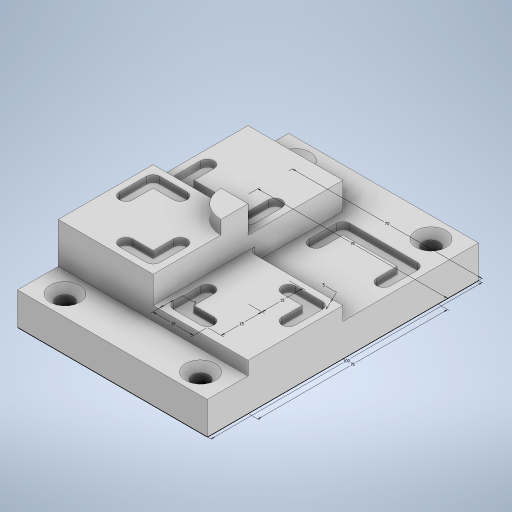
# Autodesk Inventor part: SmallTool20mm
Saved by Autodesk Inventor 2024 (Build 280153000, 153)
## iProperties
Created: 2026-02-22
Part Number: SmallTool20mm
Material: Generic
Document SubType Name: Modeling
Designer: Nathan
Density: 1 g/cm^3
Appearance: Default
Author: Nathan
Autodesk Inventor part; units mm, degrees
ref_plane "YZ Plane" through (0, 0, 0) normal (1, 0, 0) x (0, 1, 0)
ref_plane "XZ Plane" through (0, 0, 0) normal (0, 1, 0) x (-1, 0, 0)
ref_plane "XY Plane" through (0, 0, 0) normal (0, 0, 1) x (1, 0, 0)
sketch "Sketch1" plane through (0, 0, 0) normal (0, 1, 0) x (-1, 0, 0)
  line L0 (35, 50) -> (-35, 50)
  line L1 (-35, 50) -> (-35, -50)
  line L2 (-35, -50) -> (35, -50)
  line L3 (35, -50) -> (35, 50)
  line L4 (35, 50) -> (-35, -50) construction
  line L5 (-35, 50) -> (35, -50) construction
  line L6 (35, 35) -> (-35, 35)
  line L7 (-35, 35) -> (-35, -35)
  line L8 (-35, -35) -> (35, -35)
  line L9 (35, -35) -> (35, 35)
  line L10 (35, 35) -> (-35, -35) construction
  line L11 (-35, 35) -> (35, -35) construction
  line L12 (0, 35) -> (0, -35)
  line L13 (35, 0) -> (-35, 0)
  line L14 (0, 0) -> (0, 15) construction
  line L15 (0, 15) -> (15, 15) construction
  line L16 (0, 0) -> (0, -15) construction
  line L17 (0, -15) -> (-15, -15) construction
  circle A0 centre (15, 15) radius 2.5
  circle A1 centre (-15, -15) radius 2.5
  dimension "d0" = 70
  dimension "d1" = 100
  dimension "d2" = 70
  dimension "d3" = 70
  dimension "d46" = 15
  dimension "d47" = 15
  dimension "d48" = 15
  dimension "d49" = 5
  dimension "d50" = 5
  constraints: 36 end point, 8 midpoint, 4 parallel, 4 point on line, 3 perpendicular, 2 centre point, 2 coincident, 2 horizontal
  measures "d0" distance of L2.end L1.end
  measures "d1" distance of L1.end L0.end
  measures "d2" distance of L8.end L7.end
  measures "d3" distance of L7.end L6.end
  measures "d46" distance of L14.start L14.end
  measures "d47" distance of L14.end L15.end
  measures "d48" distance of L14.start L16.end
  measures "d49" diameter of A0
  measures "d50" diameter of A1
extrude "Extrusion1" add sketch "Sketch1" along normal blind 12 contours L3 L6 L1 L0 | L13 L12 L8 L1 | L3 L2 L1 L8 | A1
extrude "Extrusion2" add sketch "Sketch1" along normal blind 17 contours L6 L12 L13 L1
extrude "Extrusion3" add sketch "Sketch1" along normal blind 22 contours L3 L8 L12 L13
extrude "Extrusion4" add sketch "Sketch1" along normal blind 27 contours L3 L13 L12 L6 | A0
sketch "Sketch2" plane through (0, 27, 0) normal (0, 1, 0) x (1, 0, 0)
  line L0 (35, -35) -> (-35, -35) construction
  line L1 (35, 0) -> (0, 0) construction
  line L2 (-35, -35) -> (0, -35) construction
  line L3 (0, -35) -> (0, 0) construction
  line L4 (0, 0) -> (-35, 0) construction
  line L5 (-35, 0) -> (-35, -35) construction
  line L6 (0, -35) -> (-35, 0) construction
  line L7 (0, 0) -> (-35, -35) construction
  line L8 (-5, -32.5) -> (-15, -32.5)
  line L9 (-32.5, -15) -> (-32.5, -5)
  line L10 (-30, -2.5) -> (-20, -2.5)
  line L11 (-2.5, -20) -> (-2.5, -30)
  line L12 (-2.5, -32.5) -> (-32.5, -2.5) construction
  line L13 (-32.5, -32.5) -> (-2.5, -2.5) construction
  line L14 (-15, -27.5) -> (-10, -27.5)
  line L15 (-7.5, -25) -> (-7.5, -20)
  line L16 (-20, -7.5) -> (-25, -7.5)
  line L17 (-27.5, -10) -> (-27.5, -15)
  line L18 (-27.5, -27.5) -> (-7.5, -7.5) construction
  line L19 (-7.5, -27.5) -> (-27.5, -7.5) construction
  line L20 (-5, -17.5) -> (-5, -17.5)
  line L21 (-17.5, -30) -> (-17.5, -30)
  line L22 (-30, -17.5) -> (-30, -17.5)
  line L23 (-17.5, -5) -> (-17.5, -5)
  arc A0 (-17.5, -30) -> (-15, -32.5) centre (-15, -30) ccw
  arc A1 (-15, -27.5) -> (-17.5, -30) centre (-15, -30) ccw
  arc A2 (-5, -17.5) -> (-7.5, -20) centre (-5, -20) ccw
  arc A3 (-2.5, -20) -> (-5, -17.5) centre (-5, -20) ccw
  arc A4 (-5, -32.5) -> (-2.5, -30) centre (-5, -30) ccw
  arc A5 (-32.5, -15) -> (-30, -17.5) centre (-30, -15) ccw
  arc A6 (-30, -17.5) -> (-27.5, -15) centre (-30, -15) ccw
  arc A7 (-20, -7.5) -> (-17.5, -5) centre (-20, -5) ccw
  arc A8 (-17.5, -5) -> (-20, -2.5) centre (-20, -5) ccw
  arc A9 (-30, -2.5) -> (-32.5, -5) centre (-30, -5) ccw
  line L24 (5, -32.5) -> (15, -32.5)
  line L25 (32.5, -15) -> (32.5, -5)
  line L26 (30, -2.5) -> (20, -2.5)
  line L27 (2.5, -20) -> (2.5, -30)
  line L28 (15, -27.5) -> (10, -27.5)
  line L29 (7.5, -25) -> (7.5, -20)
  line L30 (20, -7.5) -> (25, -7.5)
  line L31 (27.5, -10) -> (27.5, -15)
  arc A10 (15, -32.5) -> (17.5, -30) centre (15, -30) ccw
  arc A11 (17.5, -30) -> (15, -27.5) centre (15, -30) ccw
  arc A12 (7.5, -20) -> (5, -17.5) centre (5, -20) ccw
  arc A13 (5, -17.5) -> (2.5, -20) centre (5, -20) ccw
  arc A14 (2.5, -30) -> (5, -32.5) centre (5, -30) ccw
  arc A15 (30, -17.5) -> (32.5, -15) centre (30, -15) ccw
  arc A16 (27.5, -15) -> (30, -17.5) centre (30, -15) ccw
  arc A17 (17.5, -5) -> (20, -7.5) centre (20, -5) ccw
  arc A18 (20, -2.5) -> (17.5, -5) centre (20, -5) ccw
  arc A19 (32.5, -5) -> (30, -2.5) centre (30, -5) ccw
  line L32 (7.5, 25) -> (7.5, 20)
  arc A20 (10, 27.5) -> (7.5, 25) centre (10, 25) ccw
  line L33 (15, 27.5) -> (10, 27.5)
  arc A21 (15, 27.5) -> (17.5, 30) centre (15, 30) ccw
  arc A22 (17.5, 30) -> (15, 32.5) centre (15, 30) ccw
  line L34 (5, 32.5) -> (15, 32.5)
  arc A23 (5, 32.5) -> (2.5, 30) centre (5, 30) ccw
  line L35 (2.5, 20) -> (2.5, 30)
  arc A24 (2.5, 20) -> (5, 17.5) centre (5, 20) ccw
  arc A25 (5, 17.5) -> (7.5, 20) centre (5, 20) ccw
  line L36 (-32.5, 15) -> (-32.5, 5)
  line L37 (-30, 2.5) -> (-20, 2.5)
  line L38 (-20, 7.5) -> (-25, 7.5)
  line L39 (-27.5, 10) -> (-27.5, 15)
  arc A26 (-30, 17.5) -> (-32.5, 15) centre (-30, 15) ccw
  arc A27 (-27.5, 15) -> (-30, 17.5) centre (-30, 15) ccw
  arc A28 (-27.5, 10) -> (-25, 7.5) centre (-25, 10) ccw
  arc A29 (-17.5, 5) -> (-20, 7.5) centre (-20, 5) ccw
  arc A30 (-20, 2.5) -> (-17.5, 5) centre (-20, 5) ccw
  arc A31 (-32.5, 5) -> (-30, 2.5) centre (-30, 5) ccw
  line L40 (-35, 50) -> (-35, 35) construction
  line L41 (35, -35) -> (35, 0) construction
  line L42 (-35, 35) -> (35, -35) construction
  line L43 (-10, -27.5) -> (-7.5, -27.5)
  line L44 (-7.5, -25) -> (-7.5, -27.5)
  line L45 (-27.5, -10) -> (-27.5, -7.5)
  line L46 (-27.5, -7.5) -> (-25, -7.5)
  line L47 (10, -27.5) -> (7.5, -27.5)
  line L48 (7.5, -27.5) -> (7.5, -25)
  line L49 (25, -7.5) -> (27.5, -7.5)
  line L50 (27.5, -7.5) -> (27.5, -10)
  point P0 (-17.5, -17.5)
  point P1 (-17.5, -17.5)
  point P2 (-7.5, -17.5)
  point P3 (-17.5, -27.5)
  point P4 (-17.5, -32.5)
  dimension "d12" = 30
  dimension "d13" = 30
  dimension "d16" = 15
  dimension "d17" = 5
  dimension "d18" = 10
  dimension "d19" = 10
  dimension "d20" = 2.5
  constraints: 94 end point, 68 symmetric about line, 64 point on circle, 32 centre point, 20 tangent, 14 point on line, 9 equal radius, 7 horizontal, 7 parallel, 7 perpendicular, 6 midpoint, 20 other
  measures "d12" distance of L12.end L13.end
  measures "d13" distance of L13.start L12.end
  measures "d16" distance of point (-17.5, -32.5) L12.start
  measures "d17" distance of point (-17.5, -27.5) point (-17.5, -32.5)
  measures "d18" distance of point (-17.5, -27.5) L19.start
  measures "d19" distance of point (-7.5, -17.5) L19.start
  measures "d20" radius of A0
fillet "Fillet1" radius 2.5 1 edges at (0, 14.5, 0)
extrude "Extrusion5" cut sketch "Sketch2" against normal blind 2.5 contours L8 A0 A1 L14 L43 L44 L15 A2 A3 L11 A4 | L9 A9 L10 A8 A7 L16 L46 L45 L17 A6 A5
extrude "Extrusion6" cut sketch "Sketch2" against normal blind 12.5 contours A14 L27 A13 A12 L29 L48 L47 L28 A11 A10 L24 | A15 A16 L31 L50 L49 L30 A17 A18 L26 A19 L25
sketch "Sketch3" plane through (0, 22, 0) normal (0, 1, 0) x (1, 0, 0)
  line L0 (0, 0) -> (0, 35) construction
  line L1 (-35, 50) -> (-35, -50) construction
  line L2 (0, 35) -> (-35, 35) construction
  line L3 (-35, 35) -> (-35, 0) construction
  line L4 (-35, 0) -> (0, 0) construction
  line L5 (0, 0) -> (0, 35) construction
  line L6 (-35, 35) -> (0, 0) construction
  line L7 (0, 35) -> (-35, 0) construction
  line L8 (-32.5, 15) -> (-32.5, 5)
  line L9 (-30, 2.5) -> (-5, 2.5)
  line L10 (-2.5, 5) -> (-2.5, 15)
  line L11 (-2.5, 32.5) -> (-32.5, 2.5) construction
  line L12 (-32.5, 32.5) -> (-2.5, 2.5) construction
  line L13 (-25, 7.5) -> (-10, 7.5)
  line L14 (-7.5, 10) -> (-7.5, 15)
  line L15 (-27.5, 15) -> (-27.5, 10)
  line L16 (-27.5, 7.5) -> (-7.5, 27.5) construction
  line L17 (-7.5, 7.5) -> (-27.5, 27.5) construction
  line L18 (-30, 17.5) -> (-30, 17.5)
  line L19 (-5, 17.5) -> (-5, 17.5)
  arc A0 (-30, 17.5) -> (-32.5, 15) centre (-30, 15) ccw
  arc A1 (-27.5, 15) -> (-30, 17.5) centre (-30, 15) ccw
  arc A2 (-5, 17.5) -> (-7.5, 15) centre (-5, 15) ccw
  arc A3 (-2.5, 15) -> (-5, 17.5) centre (-5, 15) ccw
  arc A4 (-5, 2.5) -> (-2.5, 5) centre (-5, 5) ccw
  arc A5 (-32.5, 5) -> (-30, 2.5) centre (-30, 5) ccw
  line L20 (35, 35) -> (0, 0) construction
  line L21 (0, 35) -> (35, 0) construction
  line L22 (32.5, 15) -> (32.5, 5)
  line L23 (30, 2.5) -> (5, 2.5)
  line L24 (2.5, 5) -> (2.5, 15)
  line L25 (2.5, 32.5) -> (32.5, 2.5) construction
  line L26 (32.5, 32.5) -> (2.5, 2.5) construction
  line L27 (25, 7.5) -> (10, 7.5)
  line L28 (7.5, 10) -> (7.5, 15)
  line L29 (27.5, 15) -> (27.5, 10)
  line L30 (27.5, 7.5) -> (7.5, 27.5) construction
  line L31 (7.5, 7.5) -> (27.5, 27.5) construction
  line L32 (30, 17.5) -> (30, 17.5)
  line L33 (5, 17.5) -> (5, 17.5)
  arc A6 (32.5, 15) -> (30, 17.5) centre (30, 15) ccw
  arc A7 (30, 17.5) -> (27.5, 15) centre (30, 15) ccw
  arc A8 (7.5, 15) -> (5, 17.5) centre (5, 15) ccw
  arc A9 (5, 17.5) -> (2.5, 15) centre (5, 15) ccw
  arc A10 (2.5, 5) -> (5, 2.5) centre (5, 5) ccw
  arc A11 (30, 2.5) -> (32.5, 5) centre (30, 5) ccw
  arc A12 (25, 7.5) -> (27.5, 10) centre (25, 10) ccw
  arc A13 (7.5, 10) -> (10, 7.5) centre (10, 10) ccw
  line L34 (0, 17.5) -> (35, 17.5) construction
  line L35 (35, 0) -> (35, 50) construction
  line L36 (2.5, 30) -> (2.5, 20)
  line L37 (27.5, 20) -> (27.5, 25)
  line L38 (35, 0) -> (0, 35) construction
  line L39 (25, 27.5) -> (10, 27.5)
  line L40 (30, 32.5) -> (5, 32.5)
  arc A14 (32.5, 30) -> (30, 32.5) centre (30, 30) ccw
  line L41 (32.5, 20) -> (32.5, 30)
  arc A15 (27.5, 20) -> (30, 17.5) centre (30, 20) ccw
  arc A16 (30, 17.5) -> (32.5, 20) centre (30, 20) ccw
  line L42 (7.5, 25) -> (7.5, 20)
  arc A17 (5, 32.5) -> (2.5, 30) centre (5, 30) ccw
  arc A18 (5, 17.5) -> (7.5, 20) centre (5, 20) ccw
  arc A19 (2.5, 20) -> (5, 17.5) centre (5, 20) ccw
  line L43 (-27.5, 10) -> (-27.5, 7.5)
  line L44 (-27.5, 7.5) -> (-25, 7.5)
  line L45 (-10, 7.5) -> (-7.5, 7.5)
  line L46 (-7.5, 7.5) -> (-7.5, 10)
  line L47 (7.5, 25) -> (7.5, 27.5)
  line L48 (7.5, 27.5) -> (10, 27.5)
  line L49 (25, 27.5) -> (27.5, 27.5)
  line L50 (27.5, 27.5) -> (27.5, 25)
  point P0 (-17.5, 17.5)
  point P1 (17.5, 17.5)
  dimension "d26" = 30
  dimension "d30" = 2.5
  constraints: 96 end point, 52 symmetric about line, 40 point on circle, 25 point on line, 20 centre point, 12 tangent, 7 equal length, 7 midpoint, 5 equal radius, 5 perpendicular, 3 horizontal, 1 vertical, 12 other
  measures "d26" distance of L12.end L11.end
  measures "d30" radius of A0
extrude "Extrusion7" cut sketch "Sketch3" against normal blind 2.5 contours A0 A1 L15 L43 L44 L13 L45 L46 L14 A2 A3 L10 A4 L9 A5 L8
extrude "Extrusion8" cut sketch "Sketch3" against normal blind 12.5 contours A15 L37 L50 L49 L39 L48 L47 L42 A18 A19 L36 A17 L40 A14 L41 A16
sketch "Sketch5" plane through (0, 12, 0) normal (0, 1, 0) x (1, 0, 0)
  line L0 (-35, -50) -> (35, -50) construction
  line L1 (-35, -50) -> (-35, -42.5) construction
  line L2 (-35, 50) -> (-35, -50) construction
  line L3 (-35, -42.5) -> (34.9391, -42.5) construction
  line L4 (-35, 50) -> (-35, 35) construction
  line L5 (-35, 42.5) -> (35, 42.5) construction
  line L6 (35, 0) -> (35, 50) construction
  line L7 (0, 42.5) -> (-25, 42.5) construction
  line L8 (-25, 42.5) -> (25, 42.5) construction
  line L9 (25, 42.5) -> (25, -42.5) construction
  line L10 (25, -42.5) -> (-25, -42.5) construction
  point P0 (0, 0)
  dimension "d35" = 7.5
  dimension "d36" = 25
  dimension "d37" = 50
  dimension "d38" = 50
  constraints: 14 end point, 6 point on line, 2 midpoint, 2 perpendicular, 1 horizontal
  measures "d35" distance of L0.start L1.end
  measures "d36" distance of L7.start L7.end
  measures "d37" distance of L7.end L8.end
  measures "d38" distance of L9.end L10.end
hole "Hole1" at (-25, 12, 42.5) at (-25, 12, -42.5) at (25, 12, -42.5) at (25, 12, 42.5) direction (0, -1, 0) diameter 6.1 end through all countersink diameter 11 countersink angle 90 clearance for "Countersunk Flat Head Screw ISO 2009/7046" size "M6" standard "ISO"
sketch "Sketch6" plane through (0, 27, 0) normal (0, 1, 0) x (1, 0, 0)
  line L0 (-35, 0) -> (0, 0) projected
  arc A0 (-10, 0) -> (0, -10) centre (0, 0) ccw
  line L1 (0, -10) -> (0, 0)
  line L2 (-10, 0) -> (0, 0)
  dimension "d54" = 10
  constraints: 4 end point, 2 point on circle, 1 centre point, 1 coincident, 1 collinear, 1 point on line, 1 vertical
  measures "d54" radius of A0
extrude "Extrusion10" add sketch "Sketch6" along normal blind 5
sketch "Sketch7" plane through (0, 0, 0) normal (0, -1, 0) x (1, 0, 0)
  circle A0 centre (25, -42.5) radius 3.05 construction
  line L0 (-25, 42.5) -> (25, 42.5) construction
  line L1 (25, 42.5) -> (25, -42.5) construction
  line L2 (25, -42.5) -> (-25, -42.5) construction
  line L3 (-25, -42.5) -> (-25, 42.5) construction
  line L4 (-25, 42.5) -> (25, -42.5) construction
  line L5 (25, 42.5) -> (-25, -42.5) construction
  point P0 (0, 0)
  constraints: 12 end point, 2 midpoint, 2 parallel, 1 horizontal, 1 perpendicular
extrude "Extrusion11" cut sketch "Sketch1" along normal blind 11 contours A0 | A1
body "Solid1"
